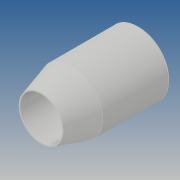
# Autodesk Inventor part: cardridge
Saved by Autodesk Inventor 2019 (Build 230136000, 136)
## iProperties
Created: 2019-03-08
Part Number: cardridge
Material: Générique
Document SubType Name: Modeling
Designer: Theo
Density: 1 g/cm^3
Appearance: Par défaut
Author: Theo
Autodesk Inventor part; units mm, degrees
ref_plane "YZ Plane" through (0, 0, 0) normal (1, 0, 0) x (0, 1, 0)
ref_plane "XZ Plane" through (0, 0, 0) normal (0, 1, 0) x (-1, 0, 0)
ref_plane "XY Plane" through (0, 0, 0) normal (0, 0, 1) x (1, 0, 0)
sketch "Esquisse1" plane through (0, 0, 0) normal (1, 0, 0) x (0, 1, 0)
  line L0 (6.55, -1) -> (6.25, -1)
  line L1 (6.25, -1) -> (6.25, -20)
  line L2 (0, 0) -> (0, -28.3478)
  line L3 (6.55, -1) -> (9.25, -10)
  line L4 (6.55, -1) -> (6.25, 0) construction
  line L5 (9.25, -10) -> (9.25, -30)
  line L6 (6.25, -20) -> (7.25, -25)
  line L7 (7.25, -25) -> (7.25, -30)
  line L8 (7.25, -30) -> (9.25, -30)
  dimension "d0" = 12.5
  dimension "d1" = 1
  dimension "d2" = 3
  dimension "d3" = 10
  dimension "d4" = 2
  dimension "d5" = 30
  dimension "d6" = 5
  dimension "d7" = 5
  dimension "d9" = 18.5
  constraints: 18 end point, 4 vertical, 2 horizontal, 1 collinear, 1 horizontal alignment, 1 vertical alignment
  measures "d0" diameter of L1 L2
  measures "d1" distance of L0.end L4.end
  measures "d2" distance between parallel lines of L5 L1
  measures "d3" vertical distance of L3.end L4.end
  measures "d4" distance of L7.end L5.end
  measures "d5" vertical distance of L5.end L4.end
  measures "d6" distance of L6.end L7.end
  measures "d7" vertical distance of L1.end L6.end
  measures "d9" diameter of L5 L2
revolve "Révolution1" add sketch "Esquisse1" angle 360 about axis through (0, 0, 0) along (0, 0, -1)
chamfer "Chanfrein1" distance 0.4 angle 45 2 edges at (0, -7.25, -30) (0, -9.25, -30)
